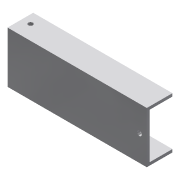
# Autodesk Inventor part: U profil
Saved by Autodesk Inventor 2015 (Build 190159000, 159)
## iProperties
Created: 2015-01-07
Part Number: U profil
Material: Všeobecné
Document SubType Name: Modeling
Designer: Michal
Density: 1 g/cm^3
Appearance: Hliník – leštěný
Author: Michal
Autodesk Inventor part; units mm, degrees
ref_plane "YZ Plane" through (0, 0, 0) normal (1, 0, 0) x (0, 1, 0)
ref_plane "XZ Plane" through (0, 0, 0) normal (0, 1, 0) x (-1, 0, 0)
ref_plane "XY Plane" through (0, 0, 0) normal (0, 0, 1) x (1, 0, 0)
sketch "Náčrt1" plane through (0, 0, 0) normal (1, 0, 0) x (0, 1, 0)
  line L0 (0, 0) -> (70, 0)
  line L1 (70, 0) -> (70, -8)
  line L2 (70, -8) -> (8, -8)
  line L3 (8, -8) -> (8, -132)
  line L4 (8, -132) -> (70, -132)
  line L5 (70, -132) -> (70, -140)
  line L6 (70, -140) -> (0, -140)
  line L7 (0, -140) -> (0, 0)
  dimension "d20" = 140
  dimension "d41" = 8
  dimension "d42" = 8
  dimension "d43" = 124
  dimension "d44" = 70
  dimension "d45" = 70
  dimension "d46" = 62
  constraints: 16 end point, 4 perpendicular, 2 point on line, 1 horizontal
  measures "d20" distance of L6.end L0.start
  measures "d41" distance of L4.end L5.end
  measures "d42" distance of L0.end L1.end
  measures "d43" distance of L2.end L3.end
  measures "d44" distance of L0.start L0.end
  measures "d45" distance of L5.end L6.end
  measures "d46" distance of L3.end L4.end
extrude "Vysunutí1" add sketch "Náčrt1" along normal blind 380
sketch "Náčrt7" plane through (0, 8, -8) normal (0, 1, 0) x (1, 0, 0)
  circle A0 centre (360, 62) radius 6.25
  line L0 (0, -8) -> (380, -8) projected
  line L1 (380, -8) -> (380, 132) projected
  dimension "d47" = 12.5
  dimension "d48" = 70
  dimension "d49" = 20
  constraints: 1 centre point
  measures "d47" diameter of A0
  measures "d48" distance from line of L0 A0.centre
  measures "d49" distance from line of L1 A0.centre
extrude "Vysunutí6" cut sketch "Náčrt7" against normal through all
sketch "Náčrt8" plane through (0, 0, 0) normal (0, 0, 1) x (1, 0, 0)
  line L0 (0, 0) -> (0, 70) projected
  line L1 (0, 0) -> (380, 0) projected
  line L2 (380, 70) -> (380, 0) projected
  line L3 (0, 70) -> (380, 70) projected
  circle A0 centre (23, 40) radius 6.25
  dimension "d52" = 12.5
  dimension "d53" = 40
  dimension "d54" = 357
  constraints: 1 centre point
  measures "d52" diameter of A0
  measures "d53" distance from line of L1 A0.centre
  measures "d54" distance from line of L2 A0.centre
extrude "Vysunutí7" cut sketch "Náčrt8" against normal through all contours A0
